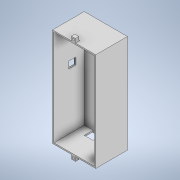
# Autodesk Inventor part: basecaixa
Saved by Autodesk Inventor 2022 (Build 260153000, 153)
## iProperties
Created: 2024-03-03
Part Number: basecaixa
Material: Genérico
Document SubType Name: Modeling
Designer: Daniel
Density: 1 g/cm^3
Appearance: Padrão
Author: Daniel
Autodesk Inventor part; units mm, degrees
ref_plane "YZ Plane" through (0, 0, 0) normal (1, 0, 0) x (0, 1, 0)
ref_plane "XZ Plane" through (0, 0, 0) normal (0, 1, 0) x (-1, 0, 0)
ref_plane "XY Plane" through (0, 0, 0) normal (0, 0, 1) x (1, 0, 0)
sketch "Esboço1" plane through (0, 0, 0) normal (0, 0, 1) x (1, 0, 0)
  line L0 (0, 0) -> (60, 0)
  line L1 (60, 0) -> (60, 110)
  line L2 (60, 110) -> (0, 110)
  line L3 (0, 110) -> (0, 0)
  line L4 (62, 112) -> (62, -2)
  line L5 (62, -2) -> (-2, -2)
  line L6 (-2, -2) -> (-2, 112)
  line L7 (-2, 112) -> (62, 112)
  dimension "d0" = 60
  dimension "d1" = 110
  dimension "d2" = 2
  constraints: 16 end point, 4 parallel, 2 perpendicular, 1 horizontal, 3 other
  measures "d0" distance of L2.end L1.end
  measures "d1" distance of L0.end L1.end
  measures "d2" distance between parallel lines of L1 L4
extrude "Extrusão1" add sketch "Esboço1" along normal blind 2 contours L3 L2 L1 L0 | L4 L5 L6 L7
sketch "Esboço2" plane through (0, 0, 2) normal (0, 0, 1) x (1, 0, 0)
  line L0 (62, 112) -> (-2, 112) projected
  line L1 (-2, 112) -> (-2, -2) projected
  line L2 (62, -2) -> (62, 112) projected
  line L3 (-2, -2) -> (62, -2) projected
  line L4 (0, 0) -> (0, 110)
  line L5 (0, 110) -> (60, 110)
  line L6 (60, 110) -> (60, 0)
  line L7 (60, 0) -> (0, 0)
  point P0 (0, 0)
  dimension "d5" = 2
  constraints: 8 end point, 3 other
  measures "d5" distance between parallel lines of L1 L4
extrude "Extrusão2" add sketch "Esboço2" along normal blind 45
sketch "Esboço3" plane through (-2, -2, 0) normal (0, -1, 0) x (1, 0, 0)
  line L0 (47, 5) -> (57, 5)
  line L1 (57, 5) -> (57, 15)
  line L2 (57, 15) -> (47, 15)
  line L3 (47, 15) -> (47, 5)
  line L4 (0, 0) -> (64, 0) projected
  line L5 (64, 0) -> (64, 47) projected
  point P0 (2, 0)
  dimension "d8" = 10
  dimension "d9" = 10
  dimension "d10" = 5
  dimension "d11" = 7
  constraints: 8 end point, 2 parallel, 1 horizontal, 1 perpendicular
  measures "d8" distance of L0.end L1.end
  measures "d9" distance of L1.end L2.end
  measures "d10" distance between parallel lines of L4 L0
  measures "d11" distance between parallel lines of L5 L1
extrude "Extrusão3" cut sketch "Esboço3" against normal blind 38
sketch "Esboço11" plane through (-2, 112, 0) normal (0, 1, 0) x (1, 0, 0)
  line L0 (64, 0) -> (64, -47) projected
  line L1 (0, 0) -> (64, 0)
  line L2 (64, 0) -> (64, -2)
  line L3 (64, -2) -> (0, -2)
  line L4 (0, -2) -> (0, 0)
  line L5 (64, 0) -> (0, 0) projected
  point P0 (2, 0)
  dimension "d45" = 2
  dimension "d46" = 0
  dimension "d47" = 64
  constraints: 8 end point, 2 parallel, 1 horizontal, 1 perpendicular, 1 point on line
  measures "d45" distance of L3.end L1.start
  measures "d46" distance between parallel lines of L5 L1
  measures "d47" distance between parallel lines of L4 L0
extrude "Extrusão8" add sketch "Esboço11" along normal blind 32
sketch "Esboço18" plane through (-2, 112, 2) normal (0, 0, 1) x (1, 0, 0)
  line L0 (0, 0) -> (64, 0) projected
  line L1 (64, 32) -> (64, 0) projected
  line L2 (0, 32) -> (64, 32) projected
  line L3 (0, 0) -> (0, 32) projected
  line L4 (0, -114) -> (0, 0) projected
  line L5 (64, -114) -> (0, -114) projected
  line L6 (64, 0) -> (64, -114) projected
  line L7 (2, -112) -> (62, -112) projected
  line L8 (62, -112) -> (62, -2) projected
  line L9 (62, -2) -> (2, -2) projected
  line L10 (2, -2) -> (2, -112) projected
  line L11 (62, 0) -> (62, 30)
  line L12 (62, 30) -> (2, 30)
  line L13 (2, 30) -> (2, 0)
  dimension "d89" = 2
  constraints: 6 end point, 2 other
  measures "d89" distance between parallel lines of L2 L12
extrude "Extrusão15" add sketch "Esboço18" along normal blind 45 contours L3 L2 L1 L0 L11 L12 L13
sketch "Esboço20" plane through (-2, -2, 0) normal (-1, 0, 0) x (0, 0, 1)
  line L0 (25, 86) -> (15, 86)
  line L1 (15, 86) -> (15, 96)
  line L2 (15, 96) -> (25, 96)
  line L3 (25, 96) -> (25, 86)
  line L4 (0, 146) -> (47, 146) projected
  line L5 (0, 146) -> (0, 0) projected
  point P0 (0, 2)
  dimension "d101" = 10
  dimension "d102" = 10
  dimension "d103" = 50
  dimension "d104" = 15
  constraints: 8 end point, 2 parallel, 1 horizontal, 1 perpendicular
  measures "d101" distance of L0.end L1.end
  measures "d102" distance of L1.end L2.end
  measures "d103" distance between parallel lines of L4 L2
  measures "d104" distance between parallel lines of L5 L1
extrude "Extrusão17" cut sketch "Esboço20" against normal blind 2
sketch "Esboço21" plane through (-2, -2, 0) normal (0, -1, 0) x (1, 0, 0)
  line L0 (62, 47) -> (2, 47) projected
  line L1 (28, 47) -> (34, 47)
  line L2 (34, 47) -> (34, 42)
  line L3 (34, 42) -> (28, 42)
  line L4 (28, 42) -> (28, 47)
  line L5 (64, 0) -> (64, 47) projected
  point P0 (2, 0)
  dimension "d108" = 6
  dimension "d109" = 5
  dimension "d110" = 30
  constraints: 8 end point, 2 parallel, 1 horizontal, 1 perpendicular, 1 point on line
  measures "d108" distance of L2.end L3.end
  measures "d109" distance of L1.end L2.end
  measures "d110" distance between parallel lines of L5 L2
extrude "Extrusão18" add sketch "Esboço21" along normal blind 6
sketch "Esboço22" plane through (0, 0, 47) normal (0, 0, 1) x (1, 0, 0)
  circle A0 centre (29, -5) radius 1.5
  line L0 (32, -2) -> (32, -8) projected
  line L1 (32, -8) -> (26, -8) projected
  point P0 (0, 0)
  dimension "d113" = 3
  dimension "d114" = 3
  dimension "d115" = 3
  constraints: 1 centre point
  measures "d113" diameter of A0
  measures "d114" distance from line of L0 A0.centre
  measures "d115" distance from line of L1 A0.centre
extrude "Extrusão19" cut sketch "Esboço22" against normal blind 6
sketch "Esboço23" plane through (-2, 144, 0) normal (0, 1, 0) x (1, 0, 0)
  line L0 (64, 0) -> (64, -47) projected
  line L1 (64, -47) -> (0, -47) projected
  line L2 (0, -47) -> (0, 0) projected
  line L3 (0, 0) -> (64, 0) projected
  line L4 (34, -42) -> (28, -42) projected
  line L5 (28, -42) -> (28, -47) projected
  line L6 (34, -47) -> (34, -42) projected
  point P0 (2, 0)
extrude "Extrusão20" add sketch "Esboço23" along normal blind 6 contours L1 L5 L4 L6
sketch "Esboço24" plane through (0, 0, 47) normal (0, 0, 1) x (1, 0, 0)
  circle A0 centre (29, 147) radius 1.5
  line L0 (26, 150) -> (32, 150) projected
  line L1 (32, 144) -> (32, 150) projected
  point P0 (0, 0)
  dimension "d120" = 3
  dimension "d121" = 3
  dimension "d122" = 3
  constraints: 1 centre point
  measures "d120" diameter of A0
  measures "d121" distance from line of L0 A0.centre
  measures "d122" distance from line of A0.centre L1
extrude "Extrusão21" cut sketch "Esboço24" against normal blind 6
chamfer "Chanfro2" distance 1.5 angle 45 2 edges at (29, 144, 42) (29, -2, 42)
sketch "Esboço25" plane through (0, 0, 47) normal (0, 0, 1) x (1, 0, 0)
  line L0 (0, 0) -> (0, 110) projected
  line L1 (0, 110) -> (60, 110)
  line L2 (60, 110) -> (60, 112)
  line L3 (60, 112) -> (0, 112)
  line L4 (0, 112) -> (0, 110)
  constraints: 8 end point, 2 parallel, 1 horizontal, 1 perpendicular
extrude "Extrusão22" cut sketch "Esboço25" against normal blind 45
sketch "Esboço26" plane through (-2, -2, 0) normal (0, -1, 0) x (1, 0, 0)
  line L0 (15, 3) -> (28, 3)
  line L1 (28, 3) -> (28, 15)
  line L2 (28, 15) -> (15, 15)
  line L3 (15, 15) -> (15, 3)
  line L4 (0, 0) -> (0, 47) projected
  line L5 (0, 0) -> (64, 0) projected
  point P0 (2, 0)
  dimension "d130" = 13
  dimension "d131" = 12
  dimension "d132" = 15
  dimension "d133" = 3
  constraints: 8 end point, 2 parallel, 1 horizontal, 1 perpendicular
  measures "d130" distance of L1.end L2.end
  measures "d131" distance of L2.end L0.start
  measures "d132" distance between parallel lines of L4 L3
  measures "d133" distance between parallel lines of L5 L0
extrude "Extrusão23" cut sketch "Esboço26" against normal blind 10
